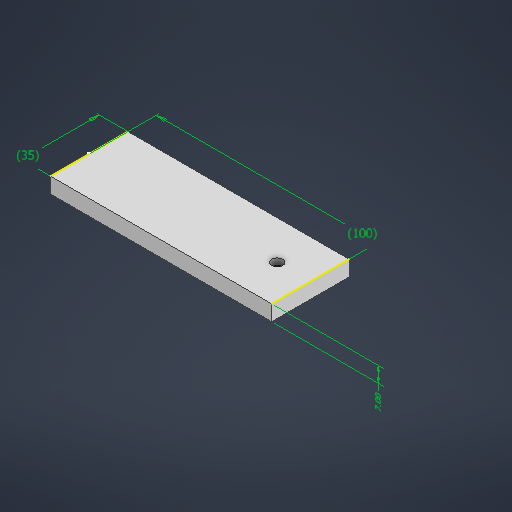
# Autodesk Inventor part: piano di carico
Saved by Autodesk Inventor 2026.2 (Build 302298000, 298)
## iProperties
Created: 2026-01-19
Part Number: piano di carico
Material: Generic
Document SubType Name: Modeling
Designer: ASUS
Density: 1 g/cm^3
Appearance: Default
Author: ASUS
Autodesk Inventor part; units mm, degrees
ref_plane "YZ Plane" through (0, 0, 0) normal (1, 0, 0) x (0, 1, 0)
ref_plane "XZ Plane" through (0, 0, 0) normal (0, 1, 0) x (-1, 0, 0)
ref_plane "XY Plane" through (0, 0, 0) normal (0, 0, 1) x (1, 0, 0)
sketch "Sketch1" plane through (0, 0, 0) normal (0, 1, 0) x (-1, 0, 0)
  line L0 (0, 0) -> (-100, 0)
  line L1 (-100, 0) -> (-100, 35)
  line L2 (-100, 35) -> (0, 35)
  line L3 (0, 35) -> (0, 0)
  dimension "d0" = 100
  dimension "d1" = 35
  constraints: 8 end point, 2 parallel, 1 horizontal, 1 perpendicular
  measures "d0" distance of L1.end L2.end
  measures "d1" distance of L0.end L1.end
extrude "Extrusion1" add sketch "Sketch1" along normal blind 7
sketch "Sketch2" plane through (0, 7, 0) normal (0, 1, 0) x (1, 0, 0)
  line L0 (0, 0) -> (0, -35) projected
  line L1 (100, -35) -> (100, 0) projected
  circle A0 centre (85, -17.5) radius 1.5
  line L2 (0, -35) -> (100, -35) projected
  line L3 (50, -35) -> (50, 0)
  line L4 (100, 0) -> (0, 0) projected
  circle A1 centre (85, -17.5) radius 2.5
  point P0 (0, -17.5)
  dimension "d6" = 3
  dimension "d8" = 5
  constraints: 3 midpoint, 2 centre point, 2 end point, 1 coincident
  measures "d6" diameter of A0
  measures "d8" diameter of A1
extrude "Extrusion2" cut sketch "Sketch2" against normal blind 3 contours A0 | A1
sketch "Sketch3" plane through (85, 4, 17.5) normal (0, 1, 0) x (1, 0, 0)
  circle A0 centre (0, 0) radius 1.6
  point P0 (-85, 17.5)
  dimension "d11" = 3.2
  constraints: 1 centre point
  measures "d11" diameter of A0
extrude "Extrusion3" cut sketch "Sketch3" against normal blind 4
sketch "Sketch4" plane through (0, 7, 0) normal (0, 1, 0) x (1, 0, 0)
  line L0 (100, -35) -> (100, 0) projected
  line L1 (0, 0) -> (0, -35) projected
  point P0 (0, -17.5)
  dimension "d14" = 100
  dimension "d15" = 35
  constraints: 1 midpoint
  measures "d14" distance from line of L0 point (0, -17.5)
  measures "d15" distance of L1.end L1.start
body "Solid1"
